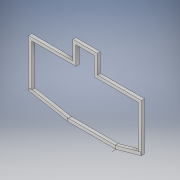
# Autodesk Inventor part: Buste2-2
Saved by Autodesk Inventor 2018 (Build 220112000, 112)
## iProperties
Created: 2018-02-13
Part Number: Buste2-2
Material: Generic
Document SubType Name: Modeling
Designer: Lilia
Density: 1 g/cm^3
Appearance: Default
Author: Lilia
Autodesk Inventor part; units mm, degrees
ref_plane "YZ Plane" through (0, 0, 0) normal (1, 0, 0) x (0, 1, 0)
ref_plane "XZ Plane" through (0, 0, 0) normal (0, 1, 0) x (-1, 0, 0)
ref_plane "XY Plane" through (0, 0, 0) normal (0, 0, 1) x (1, 0, 0)
sketch "Sketch1" plane through (0, 0, 0) normal (0, 0, 1) x (1, 0, 0)
  line L0 (-107.9, 41.925) -> (107.9, -41.925) construction
  line L1 (107.9, 41.925) -> (-107.9, -41.925) construction
  line L2 (-114.4, -47.125) -> (-114.4, 47.125)
  line L3 (114.4, 47.125) -> (114.4, -47.125)
  line L4 (114.4, -47.125) -> (-114.4, 47.125) construction
  line L5 (-114.4, -47.125) -> (114.4, 47.125) construction
  line L6 (-22.1, 47.125) -> (-22.1, 86.125)
  line L7 (-22.1, 86.125) -> (22.1, 86.125)
  line L8 (22.1, 86.125) -> (22.1, 47.125)
  line L9 (22.1, 47.125) -> (114.4, 47.125)
  line L10 (-22.1, 47.125) -> (-114.4, 47.125)
  line L11 (114.4, -47.125) -> (49.4, -75.4283)
  line L12 (-114.4, -47.125) -> (-49.4, -75.4283)
  line L13 (49.4, -75.4283) -> (-49.4, -75.4283)
  point P0 (0, 0)
  point P1 (0, 0)
  point P2 (0, 80.925)
  point P3 (0, 0)
  point P4 (0, 86.125)
  point P5 (0, 0)
  dimension "Comp" = 215.8
  dimension "Lar" = 83.85
  dimension "d10" = 215.8
  dimension "LarMaior" = 94.25
  dimension "CompMaior" = 228.8
  dimension "d20" = 39
  dimension "d21" = 44.2
  dimension "d25" = 65
  dimension "d27" = 65
  dimension "d28" = 98.8
  constraints: 28 end point, 8 midpoint, 3 equal length, 2 vertical alignment, 1 point on line
  measures "Comp" distance of L0.start L1.start
  measures "Lar" distance of L1.end L0.start
  measures "d10" distance of L0.end L1.end
  measures "LarMaior" distance of L3.start L3.end
  measures "CompMaior" distance of L2.end L3.start
  measures "d20" distance of L7.end L8.end
  measures "d21" distance of L6.end L7.end
  measures "d25" horizontal distance of L3.end L11.end
  measures "d27" horizontal distance of L2.start L12.end
  measures "d28" distance of L11.end L12.end
extrude "Extrusion1" add sketch "Sketch1" along normal blind 6.5
shell "Shell1" thickness 6.5 both sides yes removed faces 2 at (-7.3667, -34.5772, 6.5) at (-7.3667, -34.5772, 0)
sketch "Sketch2" plane through (-50.0769, -78.6783, 0) normal (-0.3992292, -0.9168512, 0) x (0.9168512, -0.3992292, 0)
  line L0 (0, 0) -> (0, -14.3)
  line L1 (-113.4763, 0) -> (-73.7013, 0) projected
  line L2 (0, -14.3) -> (-73.7013, 0)
  line L3 (-73.7013, 0) -> (0, 0)
  point P0 (14.5024, 0)
  dimension "d32" = 14.3
  constraints: 6 end point, 1 collinear, 1 vertical
  measures "d32" distance of L0.start L0.end
extrude "Extrusion2" add sketch "Sketch2" against normal blind 6.5
sketch "Sketch3" plane through (-50.0769, -78.6783, 6.5) normal (0, -1, 0) x (1, 0, 0)
  line L0 (0, -20.8002) -> (98.8, -20.8002)
  line L1 (100.2059, -6.5) -> (100.2059, -20.8002)
  line L2 (100.2059, -20.8002) -> (98.8, -20.8002)
  line L3 (0, -6.5) -> (0, 0) projected
  line L4 (0, -6.5) -> (0, -20.8002)
  line L5 (0, -6.5) -> (100.1538, -6.5) projected
  line L6 (0, -6.5) -> (100.2059, -6.5)
  line L7 (0, 0) -> (100.1538, 0) projected
  point P0 (50.0769, -6.5)
  dimension "d35" = 98.8
  constraints: 10 end point, 2 perpendicular, 1 horizontal, 1 parallel, 1 vertical
  measures "d35" distance of L0.start L0.end
extrude "Extrusion3" add sketch "Sketch3" against normal blind 6.5
sketch "Sketch4" plane through (117.65, -49.2546, 0) normal (0.3992292, -0.9168512, 0) x (0.9168512, 0.3992292, 0)
  line L0 (-165.5274, -14.3002) -> (-73.6535, -14.3002) projected
  line L1 (0, 0) -> (0, 6.5) projected
  line L2 (-73.6535, -14.3002) -> (0, 0)
  line L3 (0, 0) -> (-73.6535, 0)
  line L4 (-73.6535, 0) -> (-73.6535, -14.3002)
  point P0 (-88.2037, 0)
  constraints: 6 end point, 2 perpendicular
extrude "Extrusion4" add sketch "Sketch4" against normal blind 6.5
sketch "Sketch5" plane through (-50.0769, -78.6783, 6.5) normal (0, -1, 0) x (1, 0, 0)
  line L0 (0, -20.8) -> (0, 0) projected
  line L1 (100.2009, 0) -> (0, 0)
  line L2 (0, 0) -> (0, -14.3951)
  line L3 (0, -14.3951) -> (100.2009, -14.3951)
  line L4 (100.2009, -14.3951) -> (100.2009, 0)
  point P0 (50.0769, -6.5)
  constraints: 8 end point, 2 parallel, 1 horizontal, 1 perpendicular, 1 point on line
extrude "Extrusion5" cut sketch "Sketch5" against normal blind 6.5
sketch "Sketch6" plane through (-117.65, -49.2546, 0) normal (-0.3992292, -0.9168512, 0) x (0.9168512, -0.3992292, 0)
  line L0 (73.7013, -14.3) -> (73.7013, -7.8951) projected
  line L1 (0, 0) -> (0, 6.5) projected
  line L2 (73.7013, -7.8951) -> (0, 6.5)
  line L3 (0, 6.5) -> (73.7013, 6.5)
  line L4 (73.7013, 6.5) -> (73.7013, -7.8951)
  point P0 (88.2037, 0)
  constraints: 6 end point, 2 perpendicular
extrude "Extrusion6" cut sketch "Sketch6" against normal blind 6.5
sketch "Sketch8" plane through (50.129, -78.6556, -14.2985) normal (0.3992292, -0.9168512, 0) x (0.9168512, 0.3992292, 0)
  line L0 (-0.0136, 6.4034) -> (-91.8829, 6.4034) projected
  line L1 (-0.0054, 20.7985) -> (73.6445, 20.7985) projected
  line L2 (-0.0136, 6.4034) -> (73.6445, 20.7985)
  line L3 (73.6445, 20.7985) -> (-0.0136, 20.7985)
  line L4 (69.3853, 20.7985) -> (1.2969, 20.7985) projected
  line L5 (-0.0136, 20.7985) -> (-0.0136, 6.4034)
  line L6 (0, 0) -> (0, 14.2985) projected
  point P0 (-14.5592, 14.2985)
  constraints: 6 end point, 1 collinear, 1 parallel
extrude "Extrusion7" cut sketch "Sketch8" against normal blind 6.5
body "Solid1"
